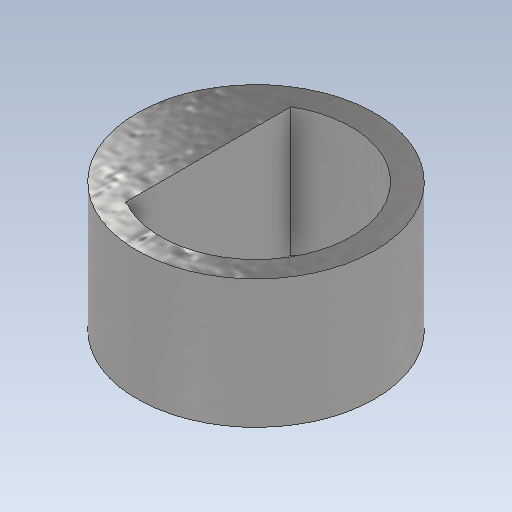
# Autodesk Inventor part: potentiometerspinny
Saved by Autodesk Inventor 2020 (Build 240168000, 168)
## iProperties
Created: 2020-01-18
Part Number: potentiometerspinny
Material: Generic
Document SubType Name: Modeling
Designer: sami_
Density: 1 g/cm^3
Appearance: Galvanized
Author: sami_
Autodesk Inventor part; units mm, degrees
ref_plane "YZ Plane" through (0, 0, 0) normal (1, 0, 0) x (0, 1, 0)
ref_plane "XZ Plane" through (0, 0, 0) normal (0, 1, 0) x (-1, 0, 0)
ref_plane "XY Plane" through (0, 0, 0) normal (0, 0, 1) x (1, 0, 0)
sketch "Sketch1" plane through (0, 0, 0) normal (0, 1, 0) x (-1, 0, 0)
  arc A0 (1, -1.7321) -> (1, 1.7321) centre (0, 0) ccw construction
  line L0 (1, 1.7321) -> (1, -1.7321)
  circle A1 centre (0, 0) radius 2.5
  arc A2 (1, 1.7321) -> (1, -1.7321) centre (0, 0) ccw
  dimension "d0" = 4
  dimension "d1" = 3
  dimension "d2" = 5
  constraints: 4 point on circle, 3 centre point, 2 coincident, 2 end point, 1 vertical
  measures "d0" diameter of A0
  measures "d2" diameter of A1
extrude "Extrusion1" add sketch "Sketch1" along normal blind 2.7
body "Solid1"
